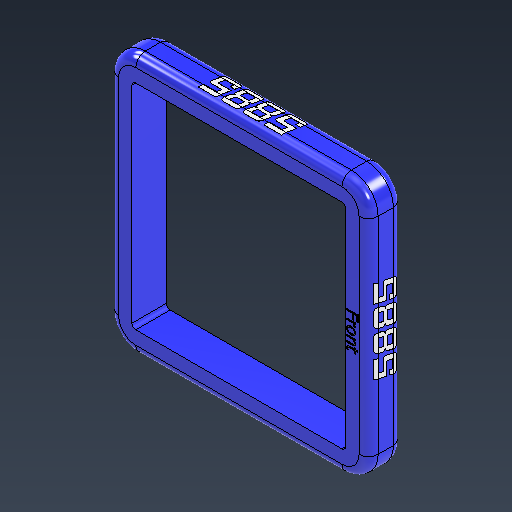
# Autodesk Inventor part: Bumpers
Saved by Autodesk Inventor 2026 (Build 300175050, 175E)
## iProperties
Created: 2026-01-21
Part Number: Bumpers
Material: Spruce
Document SubType Name: Modeling
Designer: Jthib
Mass: 10098.2 g
Surface Area: 10794.9 cm^2
Volume: 25245.5 cm^3
Density: 0.4 g/cm^3
Appearance: Blue - Wall Paint - Glossy
Author: Jthib
Autodesk Inventor part; units mm, degrees
ref_plane "YZ Plane" through (0, 0, 0) normal (1, 0, 0) x (0, 1, 0)
ref_plane "XZ Plane" through (0, 0, 0) normal (0, 1, 0) x (-1, 0, 0)
ref_plane "XY Plane" through (0, 0, 0) normal (0, 0, 1) x (1, 0, 0)
sketch "Sketch1" plane through (0, 0, 0) normal (0, 0, 1) x (1, 0, 0)
  line L0 (-355.6, 0) -> (-355.6, 342.9)
  line L1 (-342.9, 355.6) -> (342.9, 355.6)
  line L2 (355.6, 342.9) -> (355.6, -342.9)
  line L3 (342.9, -355.6) -> (-342.9, -355.6)
  line L4 (-355.6, -342.9) -> (-355.6, 0)
  arc A0 (-342.9, 355.6) -> (-355.6, 342.9) centre (-342.9, 342.9) ccw
  arc A1 (355.6, 342.9) -> (342.9, 355.6) centre (342.9, 342.9) ccw
  arc A2 (342.9, -355.6) -> (355.6, -342.9) centre (342.9, -342.9) ccw
  arc A3 (-355.6, -342.9) -> (-342.9, -355.6) centre (-342.9, -342.9) ccw
  point P0 (0, 0)
  point P1 (-355.6, 355.6)
  point P2 (355.6, 355.6)
  point P3 (355.6, -355.6)
  point P4 (-355.6, -355.6)
  dimension "d0" = 711.2
  dimension "d1" = 711.2
  dimension "d2" = 355.6
  dimension "d3" = 355.6
  dimension "d9" = 12.7
  constraints: 10 end point, 9 point on line, 8 point on circle, 8 tangent, 4 centre point, 4 perpendicular, 3 equal radius, 1 collinear, 1 vertical
  measures "d0" distance of point (355.6, 355.6) point (355.6, -355.6)
  measures "d1" distance of point (-355.6, 355.6) point (355.6, 355.6)
  measures "d2" distance from line of point (0, 0) L1
  measures "d3" distance from line of L2 point (0, 0)
  measures "d9" radius of A0
sketch "Sketch2" plane through (0, 0, 0) normal (0, 1, 0) x (-1, 0, 0)
  line L0 (400.05, 57.15) -> (355.6, 57.15)
  line L1 (355.6, 57.15) -> (355.6, -57.15)
  line L2 (355.6, -57.15) -> (400.05, -57.15)
  line L3 (431.8, -25.4) -> (431.8, 25.4)
  arc A0 (431.8, 25.4) -> (400.05, 57.15) centre (400.05, 25.4) ccw
  arc A1 (400.05, -57.15) -> (431.8, -25.4) centre (400.05, -25.4) ccw
  point P0 (0, 0)
  point P1 (431.8, 57.15)
  point P2 (355.6, 0)
  point P3 (355.6, 0)
  point P4 (355.6, 0)
  point P5 (355.6, 0)
  dimension "d4" = 114.3
  dimension "d5" = 76.2
  dimension "d6" = 31.75
  constraints: 8 end point, 4 point on circle, 4 tangent, 2 centre point, 2 parallel, 2 point on line, 1 coincident, 1 equal radius, 1 horizontal, 1 midpoint, 1 perpendicular
  measures "d4" distance of L0.end L1.end
  measures "d5" distance of point (431.8, 57.15) L0.end
  measures "d6" radius of A0
sweep "Sweep1" add profiles "Sketch2" path "Sketch1" path curves L0 A0 L1 A1 L2 A2 L3 A3 L4
sketch "Sketch3" plane through (431.8, -342.9, 25.4) normal (1, 0, 0) x (0, 0, -1)
  line L0 (-19.05, 88.9) -> (-19.05, 596.9) construction
  line L1 (-19.05, 596.9) -> (69.85, 596.9) construction
  line L2 (69.85, 596.9) -> (69.85, 88.9) construction
  line L3 (69.85, 88.9) -> (-19.05, 88.9) construction
  line L4 (-19.05, 88.9) -> (69.85, 596.9) construction
  spline S0 degree 2 poles (63.5, 216.4054) (63.5, 210.6706) (59.4791, 205.7268) (55.1945, 205.7268) knots 0 0 0 1 2 2 2
  spline S1 degree 2 poles (55.1945, 205.7268) (53.3488, 205.7268) (50.5803, 206.3201) knots 0 0 0 1 1 1
  line L5 (50.5803, 206.3201) -> (38.7152, 208.759)
  line L6 (38.7152, 208.759) -> (38.7152, 224.5132)
  line L7 (38.7152, 224.5132) -> (45.6365, 223.063)
  spline S2 degree 2 poles (45.6365, 223.063) (46.1638, 222.9311) (47.0867, 222.7993) (47.5481, 222.7993) knots 0 0 0 1 2 2 2
  spline S3 degree 2 poles (47.5481, 222.7993) (48.6687, 222.7993) (49.4597, 224.0517) (49.4597, 225.7656) knots 0 0 0 1 2 2 2
  line L8 (49.4597, 225.7656) -> (49.4597, 247.1227)
  spline S4 degree 2 poles (49.4597, 247.1227) (49.4597, 249.6934) (47.8777, 251.4073) (45.6365, 252.0005) knots 0 0 0 1 2 2 2
  line L9 (45.6365, 252.0005) -> (32.9145, 254.7031)
  spline S5 degree 2 poles (32.9145, 254.7031) (32.3213, 254.769) (31.5303, 254.9009) (31.2007, 254.9009) knots 0 0 0 1 2 2 2
  spline S6 degree 2 poles (31.2007, 254.9009) (29.1573, 254.9009) (29.1573, 252.0005) knots 0 0 0 1 1 1
  line L10 (29.1573, 252.0005) -> (29.1573, 210.8024)
  line L11 (29.1573, 210.8024) -> (-12.7, 219.7012)
  line L12 (-12.7, 219.7012) -> (-12.7, 278.3014)
  line L13 (-12.7, 278.3014) -> (1.8676, 275.2692)
  line L14 (1.8676, 275.2692) -> (1.8676, 232.7528)
  line L15 (1.8676, 232.7528) -> (16.5671, 229.5888)
  line L16 (16.5671, 229.5888) -> (16.5671, 263.536)
  spline S7 degree 2 poles (16.5671, 263.536) (16.5671, 268.1502) (20.5221, 272.3689) (24.1476, 272.3689) knots 0 0 0 1 2 2 2
  spline S8 degree 2 poles (24.1476, 272.3689) (25.6637, 272.3689) (27.3775, 271.9734) knots 0 0 0 1 1 1
  line L17 (27.3775, 271.9734) -> (50.2507, 267.1614)
  spline S9 degree 2 poles (50.2507, 267.1614) (56.9742, 265.7112) (63.5, 258.724) (63.5, 251.4073) knots 0 0 0 1 2 2 2
  line L18 (63.5, 251.4073) -> (63.5, 216.4054)
  spline S10 degree 2 poles (63.5, 289.1118) (63.5, 283.377) (59.4791, 278.3014) (55.1945, 278.3014) knots 0 0 0 1 2 2 2
  spline S11 degree 2 poles (55.1945, 278.3014) (53.3488, 278.3014) (50.5803, 278.8946) knots 0 0 0 1 1 1
  line L19 (50.5803, 278.8946) -> (32.4531, 282.7178)
  spline S12 degree 2 poles (32.4531, 282.7178) (28.1685, 283.6407) (24.4772, 289.5732) (24.1476, 293.5282) knots 0 0 0 1 2 2 2
  spline S13 degree 2 poles (24.1476, 293.5282) (23.7521, 290.2324) (20.7199, 286.6728) (17.49, 286.6728) knots 0 0 0 1 2 2 2
  spline S14 degree 2 poles (17.49, 286.6728) (16.2375, 286.6728) (14.5237, 287.0024) knots 0 0 0 1 1 1
  line L20 (14.5237, 287.0024) -> (0.2856, 290.0346)
  spline S15 degree 2 poles (0.2856, 290.0346) (-6.2401, 291.4189) (-12.7, 298.9334) (-12.7, 306.1183) knots 0 0 0 1 2 2 2
  line L21 (-12.7, 306.1183) -> (-12.7, 339.3405)
  spline S16 degree 2 poles (-12.7, 339.3405) (-12.7, 345.273) (-8.4154, 350.4804) (-4.1308, 350.4804) knots 0 0 0 1 2 2 2
  spline S17 degree 2 poles (-4.1308, 350.4804) (-1.8896, 350.4804) (0.2856, 350.019) knots 0 0 0 1 1 1
  line L22 (0.2856, 350.019) -> (14.5237, 346.9869)
  spline S18 degree 2 poles (14.5237, 346.9869) (19.2697, 345.9322) (23.6862, 340.4611) (24.1476, 336.3742) knots 0 0 0 1 2 2 2
  spline S19 degree 2 poles (24.1476, 336.3742) (24.4772, 339.6701) (27.1798, 343.8228) (30.2119, 343.8228) knots 0 0 0 1 2 2 2
  spline S20 degree 2 poles (30.2119, 343.8228) (30.7393, 343.8228) (31.8599, 343.691) (32.4531, 343.6251) knots 0 0 0 1 2 2 2
  line L23 (32.4531, 343.6251) -> (50.5803, 339.8019)
  spline S21 degree 2 poles (50.5803, 339.8019) (57.1061, 338.4176) (63.5, 331.4304) (63.5, 324.1137) knots 0 0 0 1 2 2 2
  line L24 (63.5, 324.1137) -> (63.5, 289.1118)
  spline S22 degree 2 poles (33.376, 327.7391) (32.9145, 327.8709) (32.1235, 327.8709) knots 0 0 0 1 1 1
  spline S23 degree 2 poles (32.1235, 327.8709) (30.8711, 327.8709) (29.9483, 326.3548) (29.9483, 324.4433) knots 0 0 0 1 2 2 2
  line L25 (29.9483, 324.4433) -> (29.9483, 302.9543)
  spline S24 degree 2 poles (29.9483, 302.9543) (29.9483, 300.7131) (31.3984, 298.472) (33.376, 298.1424) knots 0 0 0 1 2 2 2
  line L26 (33.376, 298.1424) -> (45.3728, 295.6375)
  spline S25 degree 2 poles (45.3728, 295.6375) (45.9661, 295.5716) (46.7571, 295.4398) (47.0867, 295.4398) knots 0 0 0 1 2 2 2
  spline S26 degree 2 poles (47.0867, 295.4398) (49.4597, 295.4398) (49.4597, 298.8016) knots 0 0 0 1 1 1
  line L27 (49.4597, 298.8016) -> (49.4597, 320.2905)
  spline S27 degree 2 poles (49.4597, 320.2905) (49.4597, 322.5317) (47.614, 324.7728) (45.3728, 325.2343) knots 0 0 0 1 2 2 2
  line L28 (45.3728, 325.2343) -> (33.376, 327.7391)
  spline S28 degree 2 poles (4.8998, 333.6057) (4.3066, 333.6716) (3.6474, 333.8035) (3.3178, 333.8035) knots 0 0 0 1 2 2 2
  spline S29 degree 2 poles (3.3178, 333.8035) (1.0766, 333.8035) (1.0766, 330.4417) knots 0 0 0 1 1 1
  line L29 (1.0766, 330.4417) -> (1.0766, 309.1505)
  spline S30 degree 2 poles (1.0766, 309.1505) (1.0766, 306.9093) (2.6587, 304.8659) (4.8998, 304.4704) knots 0 0 0 1 2 2 2
  line L30 (4.8998, 304.4704) -> (15.7102, 302.1633)
  spline S31 degree 2 poles (15.7102, 302.1633) (16.1057, 302.0974) (16.8308, 301.9656) (17.1604, 301.9656) knots 0 0 0 1 2 2 2
  spline S32 degree 2 poles (17.1604, 301.9656) (19.1379, 301.9656) (19.1379, 305.1955) knots 0 0 0 1 1 1
  line L31 (19.1379, 305.1955) -> (19.1379, 326.7503)
  spline S33 degree 2 poles (19.1379, 326.7503) (19.1379, 328.9915) (17.6218, 330.9031) (15.7102, 331.2986) knots 0 0 0 1 2 2 2
  line L32 (15.7102, 331.2986) -> (4.8998, 333.6057)
  spline S34 degree 2 poles (63.5, 361.5545) (63.5, 355.8197) (59.4791, 350.7441) (55.1945, 350.7441) knots 0 0 0 1 2 2 2
  spline S35 degree 2 poles (55.1945, 350.7441) (53.3488, 350.7441) (50.5803, 351.3374) knots 0 0 0 1 1 1
  line L33 (50.5803, 351.3374) -> (32.4531, 355.1606)
  spline S36 degree 2 poles (32.4531, 355.1606) (28.1685, 356.0834) (24.4772, 362.0159) (24.1476, 365.9709) knots 0 0 0 1 2 2 2
  spline S37 degree 2 poles (24.1476, 365.9709) (23.7521, 362.6751) (20.7199, 359.1156) (17.49, 359.1156) knots 0 0 0 1 2 2 2
  spline S38 degree 2 poles (17.49, 359.1156) (16.2375, 359.1156) (14.5237, 359.4452) knots 0 0 0 1 1 1
  line L34 (14.5237, 359.4452) -> (0.2856, 362.4773)
  spline S39 degree 2 poles (0.2856, 362.4773) (-6.2401, 363.8616) (-12.7, 371.3761) (-12.7, 378.5611) knots 0 0 0 1 2 2 2
  line L35 (-12.7, 378.5611) -> (-12.7, 411.7832)
  spline S40 degree 2 poles (-12.7, 411.7832) (-12.7, 417.7157) (-8.4154, 422.9232) (-4.1308, 422.9232) knots 0 0 0 1 2 2 2
  spline S41 degree 2 poles (-4.1308, 422.9232) (-1.8896, 422.9232) (0.2856, 422.4618) knots 0 0 0 1 1 1
  line L36 (0.2856, 422.4618) -> (14.5237, 419.4296)
  spline S42 degree 2 poles (14.5237, 419.4296) (19.2697, 418.3749) (23.6862, 412.9038) (24.1476, 408.817) knots 0 0 0 1 2 2 2
  spline S43 degree 2 poles (24.1476, 408.817) (24.4772, 412.1128) (27.1798, 416.2656) (30.2119, 416.2656) knots 0 0 0 1 2 2 2
  spline S44 degree 2 poles (30.2119, 416.2656) (30.7393, 416.2656) (31.8599, 416.1337) (32.4531, 416.0678) knots 0 0 0 1 2 2 2
  line L37 (32.4531, 416.0678) -> (50.5803, 412.2446)
  spline S45 degree 2 poles (50.5803, 412.2446) (57.1061, 410.8604) (63.5, 403.8732) (63.5, 396.5564) knots 0 0 0 1 2 2 2
  line L38 (63.5, 396.5564) -> (63.5, 361.5545)
  spline S46 degree 2 poles (33.376, 400.1818) (32.9145, 400.3137) (32.1235, 400.3137) knots 0 0 0 1 1 1
  spline S47 degree 2 poles (32.1235, 400.3137) (30.8711, 400.3137) (29.9483, 398.7976) (29.9483, 396.886) knots 0 0 0 1 2 2 2
  line L39 (29.9483, 396.886) -> (29.9483, 375.3971)
  spline S48 degree 2 poles (29.9483, 375.3971) (29.9483, 373.1559) (31.3984, 370.9147) (33.376, 370.5851) knots 0 0 0 1 2 2 2
  line L40 (33.376, 370.5851) -> (45.3728, 368.0803)
  spline S49 degree 2 poles (45.3728, 368.0803) (45.9661, 368.0144) (46.7571, 367.8825) (47.0867, 367.8825) knots 0 0 0 1 2 2 2
  spline S50 degree 2 poles (47.0867, 367.8825) (49.4597, 367.8825) (49.4597, 371.2443) knots 0 0 0 1 1 1
  line L41 (49.4597, 371.2443) -> (49.4597, 392.7332)
  spline S51 degree 2 poles (49.4597, 392.7332) (49.4597, 394.9744) (47.614, 397.2156) (45.3728, 397.677) knots 0 0 0 1 2 2 2
  line L42 (45.3728, 397.677) -> (33.376, 400.1818)
  spline S52 degree 2 poles (4.8998, 406.0484) (4.3066, 406.1144) (3.6474, 406.2462) (3.3178, 406.2462) knots 0 0 0 1 2 2 2
  spline S53 degree 2 poles (3.3178, 406.2462) (1.0766, 406.2462) (1.0766, 402.8844) knots 0 0 0 1 1 1
  line L43 (1.0766, 402.8844) -> (1.0766, 381.5933)
  spline S54 degree 2 poles (1.0766, 381.5933) (1.0766, 379.3521) (2.6587, 377.3086) (4.8998, 376.9131) knots 0 0 0 1 2 2 2
  line L44 (4.8998, 376.9131) -> (15.7102, 374.6061)
  spline S55 degree 2 poles (15.7102, 374.6061) (16.1057, 374.5401) (16.8308, 374.4083) (17.1604, 374.4083) knots 0 0 0 1 2 2 2
  spline S56 degree 2 poles (17.1604, 374.4083) (19.1379, 374.4083) (19.1379, 377.6382) knots 0 0 0 1 1 1
  line L45 (19.1379, 377.6382) -> (19.1379, 399.1931)
  spline S57 degree 2 poles (19.1379, 399.1931) (19.1379, 401.4343) (17.6218, 403.3458) (15.7102, 403.7413) knots 0 0 0 1 2 2 2
  line L46 (15.7102, 403.7413) -> (4.8998, 406.0484)
  spline S58 degree 2 poles (63.5, 434.4586) (63.5, 428.7239) (59.4791, 423.7801) (55.1945, 423.7801) knots 0 0 0 1 2 2 2
  spline S59 degree 2 poles (55.1945, 423.7801) (53.3488, 423.7801) (50.5803, 424.3734) knots 0 0 0 1 1 1
  line L47 (50.5803, 424.3734) -> (38.7152, 426.8123)
  line L48 (38.7152, 426.8123) -> (38.7152, 442.5664)
  line L49 (38.7152, 442.5664) -> (45.6365, 441.1163)
  spline S60 degree 2 poles (45.6365, 441.1163) (46.1638, 440.9844) (47.0867, 440.8526) (47.5481, 440.8526) knots 0 0 0 1 2 2 2
  spline S61 degree 2 poles (47.5481, 440.8526) (48.6687, 440.8526) (49.4597, 442.105) (49.4597, 443.8189) knots 0 0 0 1 2 2 2
  line L50 (49.4597, 443.8189) -> (49.4597, 465.1759)
  spline S62 degree 2 poles (49.4597, 465.1759) (49.4597, 467.7467) (47.8777, 469.4606) (45.6365, 470.0538) knots 0 0 0 1 2 2 2
  line L51 (45.6365, 470.0538) -> (32.9145, 472.7564)
  spline S63 degree 2 poles (32.9145, 472.7564) (32.3213, 472.8223) (31.5303, 472.9541) (31.2007, 472.9541) knots 0 0 0 1 2 2 2
  spline S64 degree 2 poles (31.2007, 472.9541) (29.1573, 472.9541) (29.1573, 470.0538) knots 0 0 0 1 1 1
  line L52 (29.1573, 470.0538) -> (29.1573, 428.8557)
  line L53 (29.1573, 428.8557) -> (-12.7, 437.7545)
  line L54 (-12.7, 437.7545) -> (-12.7, 496.3547)
  line L55 (-12.7, 496.3547) -> (1.8676, 493.3225)
  line L56 (1.8676, 493.3225) -> (1.8676, 450.8061)
  line L57 (1.8676, 450.8061) -> (16.5671, 447.642)
  line L58 (16.5671, 447.642) -> (16.5671, 481.5893)
  spline S65 degree 2 poles (16.5671, 481.5893) (16.5671, 486.2035) (20.5221, 490.4221) (24.1476, 490.4221) knots 0 0 0 1 2 2 2
  spline S66 degree 2 poles (24.1476, 490.4221) (25.6637, 490.4221) (27.3775, 490.0266) knots 0 0 0 1 1 1
  line L59 (27.3775, 490.0266) -> (50.2507, 485.2147)
  spline S67 degree 2 poles (50.2507, 485.2147) (56.9742, 483.7645) (63.5, 476.7773) (63.5, 469.4606) knots 0 0 0 1 2 2 2
  line L60 (63.5, 469.4606) -> (63.5, 434.4586)
  point P0 (25.4, 342.9)
  point P1 (25.4, 342.9)
  dimension "d2" = 355.6
  dimension "d10" = 508
  dimension "d11" = 88.9
  constraints: 2 end point, 1 coincident, 1 horizontal, 1 midpoint, 2 other
  measures "d10" distance of L0.start L0.end
  measures "d11" distance of L0.end L1.end
emboss "Emboss1" sketch "Sketch3" operation cut depth 0.254 direction (-1, 0, 0)
pattern_circular "Circular Pattern1" count 4 over 360 about axis through (0, 0, -10) along (0, 0, 1) of "Emboss1"
sketch "Sketch4" plane through (-342.9, -400.05, 57.15) normal (0, 0, 1) x (1, 0, 0)
  line L0 (698.5, 527.05) -> (698.5, 273.05) construction
  line L1 (698.5, 273.05) -> (742.95, 273.05) construction
  line L2 (742.95, 273.05) -> (742.95, 527.05) construction
  line L3 (742.95, 527.05) -> (698.5, 527.05) construction
  line L4 (698.5, 742.95) -> (698.5, 57.15) projected
  line L5 (742.95, 742.95) -> (742.95, 57.15) projected
  line L6 (735.6686, 434.1053) -> (735.6686, 451.8277)
  line L7 (735.6686, 451.8277) -> (724.924, 451.8277)
  line L8 (724.924, 451.8277) -> (724.924, 434.8464)
  line L9 (724.924, 434.8464) -> (720.4162, 434.8464)
  line L10 (720.4162, 434.8464) -> (720.4162, 451.8277)
  line L11 (720.4162, 451.8277) -> (702.0764, 451.8277)
  line L12 (702.0764, 451.8277) -> (702.0764, 456.8912)
  line L13 (702.0764, 456.8912) -> (740.1764, 456.8912)
  line L14 (740.1764, 456.8912) -> (740.1764, 434.1053)
  line L15 (740.1764, 434.1053) -> (735.6686, 434.1053)
  line L16 (725.5107, 414.7775) -> (725.5107, 415.0245)
  spline S0 degree 2 poles (725.5107, 415.0245) (725.665, 415.5802) (725.7268, 416.7844) (725.7268, 417.618) knots 0 0 0 1 2 2 2
  spline S1 degree 2 poles (725.7268, 417.618) (725.7268, 419.5631) (724.0286, 423.3917) (722.3614, 425.1207) knots 0 0 0 1 2 2 2
  line L17 (722.3614, 425.1207) -> (702.0764, 425.1207)
  line L18 (702.0764, 425.1207) -> (702.0764, 429.9372)
  line L19 (702.0764, 429.9372) -> (730.6668, 429.9372)
  line L20 (730.6668, 429.9372) -> (730.6668, 425.1207)
  line L21 (730.6668, 425.1207) -> (726.406, 425.1207)
  spline S2 degree 2 poles (726.406, 425.1207) (728.7526, 422.4963) (730.6668, 418.5751) (730.6668, 416.7226) knots 0 0 0 1 2 2 2
  spline S3 degree 2 poles (730.6668, 416.7226) (730.6668, 415.9816) (730.6051, 415.2406) (730.5124, 414.7775) knots 0 0 0 1 2 2 2
  line L22 (730.5124, 414.7775) -> (725.5107, 414.7775)
  spline S4 degree 2 poles (716.3716, 387.5455) (709.1468, 387.5455) (701.2736, 394.4925) (701.2736, 400.297) knots 0 0 0 1 2 2 2
  spline S5 degree 2 poles (701.2736, 400.297) (701.2736, 406.2559) (709.3938, 413.0793) (716.3716, 413.0793) knots 0 0 0 1 2 2 2
  spline S6 degree 2 poles (716.3716, 413.0793) (723.5346, 413.0793) (731.4696, 406.0398) (731.4696, 400.297) knots 0 0 0 1 2 2 2
  spline S7 degree 2 poles (731.4696, 400.297) (731.4696, 394.4925) (723.5655, 387.5455) (716.3716, 387.5455) knots 0 0 0 1 2 2 2
  spline S8 degree 2 poles (716.3716, 392.5164) (721.9291, 392.5164) (727.3323, 396.5611) (727.3323, 400.297) knots 0 0 0 1 2 2 2
  spline S9 degree 2 poles (727.3323, 400.297) (727.3323, 404.0329) (721.9291, 408.1084) (716.3716, 408.1084) knots 0 0 0 1 2 2 2
  spline S10 degree 2 poles (716.3716, 408.1084) (710.9684, 408.1084) (705.4109, 404.0329) (705.4109, 400.297) knots 0 0 0 1 2 2 2
  spline S11 degree 2 poles (705.4109, 400.297) (705.4109, 396.592) (710.8758, 392.5164) (716.3716, 392.5164) knots 0 0 0 1 2 2 2
  line L23 (702.0764, 360.1592) -> (702.0764, 364.9758)
  line L24 (702.0764, 364.9758) -> (718.3785, 364.9758)
  spline S12 degree 2 poles (718.3785, 364.9758) (720.3545, 364.9758) (723.7508, 365.3463) (724.7697, 365.902) knots 0 0 0 1 2 2 2
  spline S13 degree 2 poles (724.7697, 365.902) (725.8503, 366.4887) (726.9, 368.5882) (726.9, 370.3789) knots 0 0 0 1 2 2 2
  spline S14 degree 2 poles (726.9, 370.3789) (726.9, 372.1697) (724.9858, 375.9673) (723.442, 377.789) knots 0 0 0 1 2 2 2
  line L25 (723.442, 377.789) -> (702.0764, 377.789)
  line L26 (702.0764, 377.789) -> (702.0764, 382.6055)
  line L27 (702.0764, 382.6055) -> (730.6668, 382.6055)
  line L28 (730.6668, 382.6055) -> (730.6668, 377.789)
  line L29 (730.6668, 377.789) -> (727.4867, 377.789)
  spline S15 degree 2 poles (727.4867, 377.789) (729.4318, 375.6277) (731.4696, 371.4596) (731.4696, 369.113) knots 0 0 0 1 2 2 2
  spline S16 degree 2 poles (731.4696, 369.113) (731.4696, 364.914) (725.912, 360.1592) (720.6324, 360.1592) knots 0 0 0 1 2 2 2
  line L30 (720.6324, 360.1592) -> (702.0764, 360.1592)
  spline S17 degree 2 poles (701.5206, 344.7525) (701.5206, 348.6737) (705.9975, 353.0888) (710.8449, 353.0888) knots 0 0 0 1 2 2 2
  line L31 (710.8449, 353.0888) -> (726.6839, 353.0888)
  line L32 (726.6839, 353.0888) -> (726.6839, 356.3307)
  line L33 (726.6839, 356.3307) -> (730.6668, 356.3307)
  line L34 (730.6668, 356.3307) -> (730.6668, 353.0888)
  line L35 (730.6668, 353.0888) -> (738.8796, 353.0888)
  line L36 (738.8796, 353.0888) -> (738.8796, 348.2723)
  line L37 (738.8796, 348.2723) -> (730.6668, 348.2723)
  line L38 (730.6668, 348.2723) -> (730.6668, 339.4111)
  line L39 (730.6668, 339.4111) -> (726.6839, 339.4111)
  line L40 (726.6839, 339.4111) -> (726.6839, 348.2723)
  line L41 (726.6839, 348.2723) -> (713.0679, 348.2723)
  spline S18 degree 2 poles (713.0679, 348.2723) (710.9067, 348.2723) (708.5293, 348.1179) (707.5104, 347.593) knots 0 0 0 1 2 2 2
  spline S19 degree 2 poles (707.5104, 347.593) (706.615, 347.1608) (705.7197, 345.2156) (705.7197, 343.5484) knots 0 0 0 1 2 2 2
  spline S20 degree 2 poles (705.7197, 343.5484) (705.7197, 342.3751) (706.4298, 340.183) (706.6459, 339.689) knots 0 0 0 1 2 2 2
  line L42 (706.6459, 339.689) -> (706.6459, 339.4111)
  line L43 (706.6459, 339.4111) -> (702.3234, 339.4111)
  spline S21 degree 2 poles (702.3234, 339.4111) (701.9529, 340.7696) (701.5206, 343.5484) (701.5206, 344.7525) knots 0 0 0 1 2 2 2
  point P0 (342.9, 400.05)
  point P1 (742.95, 400.05)
  dimension "d2" = 355.6
  dimension "d17" = 254
  constraints: 2 midpoint, 1 collinear, 2 other
  measures "d17" distance between parallel lines of L1 L3
emboss "Emboss2" sketch "Sketch4" operation cut depth 2.54 direction (0, 0, -1)
equation "\"d0\" = d1"
equation "\"d2\" = 0.5 * d0"
equation "\"d3\" = 0.5 * d1"
body "Solid1"
